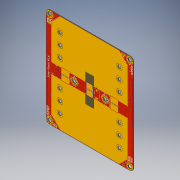
# Autodesk Inventor part: SolarPanel_PCB
Saved by Autodesk Inventor 2018 (Build 220112000, 112)
## iProperties
Created: 2018-11-29
Part Number: SolarPanel_PCB
Material: Epoxy Resin
Document SubType Name: Modeling
Designer: Bradley
Density: 1.14 g/cm^3
Appearance: Smooth - Dark Gray
Author: Bradley
Autodesk Inventor part; units mm, degrees
ref_plane "YZ Plane" through (0, 0, 0) normal (1, 0, 0) x (0, 1, 0)
ref_plane "XZ Plane" through (0, 0, 0) normal (0, 1, 0) x (-1, 0, 0)
ref_plane "XY Plane" through (0, 0, 0) normal (0, 0, 1) x (1, 0, 0)
sketch "Sketch1" plane through (0, 0, 0) normal (0, 1, 0) x (-1, 0, 0)
  line L0 (36.5, -45) -> (-36.5, -45)
  line L1 (-39.5, -42) -> (-39.5, 42)
  line L2 (-36.5, 45) -> (36.5, 45)
  line L3 (39.5, 42) -> (39.5, -42)
  line L4 (39.5, -45) -> (-39.5, 45) construction
  line L5 (-39.5, -45) -> (39.5, 45) construction
  arc A0 (39.5, 42) -> (36.5, 45) centre (36.5, 42) ccw
  arc A1 (36.5, -45) -> (39.5, -42) centre (36.5, -42) ccw
  arc A2 (-39.5, -42) -> (-36.5, -45) centre (-36.5, -42) ccw
  arc A3 (-36.5, 45) -> (-39.5, 42) centre (-36.5, 42) ccw
  circle A4 centre (36.5, 42) radius 1.65
  circle A5 centre (-36.5, 42) radius 1.65
  circle A6 centre (-36.5, -42) radius 1.65
  circle A7 centre (36.5, -42) radius 1.65
  line L6 (14, 0) -> (-14, 0) construction
  circle A8 centre (14, 0) radius 1.65
  circle A9 centre (-14, 0) radius 1.65
  point P0 (0, 0)
  point P1 (0, 0)
  dimension "d0" = 79
  dimension "d1" = 90
  dimension "d2" = 3
  dimension "d3" = 3.3
  dimension "d4" = 28
  constraints: 14 end point, 10 centre point, 8 equal radius, 8 point on circle, 8 point on line, 8 tangent, 6 coincident, 4 midpoint, 2 horizontal, 2 parallel, 1 perpendicular
  measures "d0" distance of L4.end L5.end
  measures "d1" distance of L5.end L4.start
  measures "d2" radius of A0
  measures "d3" diameter of A4
  measures "d4" distance of L6.start L6.end
extrude "Extrusion1" add sketch "Sketch1" along normal mid plane 0.6
sketch "Sketch2" plane through (0, -0.3, 0) normal (0, -1, 0) x (1, 0, 0)
  circle A0 centre (14, 0) radius 1.65 projected
  circle A1 centre (-14, 0) radius 1.65 projected
  circle A2 centre (-36.5, -42) radius 1.65 projected
  circle A3 centre (36.5, -42) radius 1.65 projected
  circle A4 centre (36.5, 42) radius 1.65 projected
  circle A5 centre (-36.5, 42) radius 1.65 projected
  line L0 (-39.5, 42) -> (-39.5, -42) projected
  arc A6 (-39.5, -42) -> (-36.5, -45) centre (-36.5, -42) ccw projected
  line L1 (-36.5, -45) -> (36.5, -45) projected
  arc A7 (36.5, -45) -> (39.5, -42) centre (36.5, -42) ccw projected
  line L2 (39.5, -42) -> (39.5, 42) projected
  arc A8 (39.5, 42) -> (36.5, 45) centre (36.5, 42) ccw projected
  line L3 (36.5, 45) -> (-36.5, 45) projected
  arc A9 (-36.5, 45) -> (-39.5, 42) centre (-36.5, 42) ccw projected
  line L4 (-39.5, 42) -> (-39.5, -42) projected
  line L5 (39.5, -42) -> (39.5, 42) projected
  line L6 (-39.5, 44.9931) -> (39.5, 44.9931) construction
  line L7 (39.5, 44.9931) -> (39.5, -44.9931) construction
  line L8 (39.5, -44.9931) -> (-39.5, -44.9931) construction
  line L9 (-39.5, -44.9931) -> (-39.5, 44.9931) construction
  point P0 (0, 0)
  point P1 (39.5, 0)
  point P2 (39.5, 0)
  point P3 (39.5, 0)
  point P4 (39.5, 0)
  point P5 (39.5, 0)
  point P6 (39.5, 0)
  constraints: 7 midpoint, 2 collinear, 2 other
decal "Decal1"
sketch "Sketch3" plane through (0, 0.3, 0) normal (0, 1, 0) x (1, 0, 0)
  circle A0 centre (14, 0) radius 1.65 projected
  circle A1 centre (-14, 0) radius 1.65 projected
  circle A2 centre (-36.5, 42) radius 1.65 projected
  circle A3 centre (36.5, 42) radius 1.65 projected
  circle A4 centre (36.5, -42) radius 1.65 projected
  circle A5 centre (-36.5, -42) radius 1.65 projected
  line L0 (-39.5, 42) -> (-39.5, -42) projected
  arc A6 (-39.5, -42) -> (-36.5, -45) centre (-36.5, -42) ccw projected
  line L1 (-36.5, -45) -> (36.5, -45) projected
  arc A7 (36.5, -45) -> (39.5, -42) centre (36.5, -42) ccw projected
  line L2 (39.5, -42) -> (39.5, 42) projected
  arc A8 (39.5, 42) -> (36.5, 45) centre (36.5, 42) ccw projected
  line L3 (36.5, 45) -> (-36.5, 45) projected
  arc A9 (-36.5, 45) -> (-39.5, 42) centre (-36.5, 42) ccw projected
  line L4 (39.5, -42) -> (39.5, 42) projected
  line L5 (39.5, -44.9829) -> (-39.5, -44.9829) construction
  line L6 (-39.5, -44.9829) -> (-39.5, 44.9829) construction
  line L7 (-39.5, 44.9829) -> (39.5, 44.9829) construction
  line L8 (39.5, 44.9829) -> (39.5, -44.9829) construction
  point P0 (0, 0)
  point P1 (39.5, 0)
  point P2 (39.5, 0)
  point P3 (39.5, 0)
  point P4 (39.5, 0)
  point P5 (39.5, 0)
  constraints: 6 midpoint, 2 collinear, 2 other
decal "Decal2"
sketch "Sketch4" plane through (0, -0.3, 0) normal (0, -1, 0) x (1, 0, 0)
  point P0 (0, 0)
  point P1 (27, -22)
  point P2 (27, 32)
  point P3 (27, 22)
  point P4 (27, 12)
  point P5 (-27, 32)
  point P6 (27, -12)
  point P7 (-27, 22)
  point P8 (-27, 12)
  point P9 (-27, -32)
  point P10 (-27, -22)
  point P11 (27, -32)
  point P12 (-27, -12)
  constraints: 12 other
hole "Hole1" at (27, -0.3, -22) at (27, -0.3, 32) at (27, -0.3, 22) at (27, -0.3, 12) at (-27, -0.3, 32) at (27, -0.3, -12) at (-27, -0.3, 22) at (-27, -0.3, 12) at (-27, -0.3, -32) at (-27, -0.3, -22) at (27, -0.3, -32) at (-27, -0.3, -12) direction (0, 1, 0) diameter 3 end through all
sketch "Sketch5" plane through (0, -0.3, 0) normal (0, -1, 0) x (1, 0, 0)
  point P0 (0, 0)
  point P1 (-12.374, -1.626)
  point P2 (-15.626, -1.626)
  point P3 (-14, -2.3)
  point P4 (-15.626, 1.626)
  point P5 (-14, 2.3)
  point P6 (-12.374, 1.626)
  point P7 (-11.7, 0)
  point P8 (-16.3, 0)
  point P9 (34.874, -40.374)
  point P10 (38.126, -43.626)
  point P11 (34.874, -43.626)
  point P12 (36.5, -39.7)
  point P13 (38.126, -40.374)
  point P14 (38.8, -42)
  point P15 (34.2, -42)
  point P16 (36.5, -44.3)
  point P17 (34.874, 40.374)
  point P18 (36.5, 39.7)
  point P19 (34.874, 43.626)
  point P20 (36.5, 44.3)
  point P21 (38.126, 43.626)
  point P22 (38.8, 42)
  point P23 (34.2, 42)
  point P24 (38.126, 40.374)
  point P25 (-34.874, 40.374)
  point P26 (-38.126, 40.374)
  point P27 (-36.5, 39.7)
  point P28 (-38.126, 43.626)
  point P29 (-36.5, 44.3)
  point P30 (-34.874, 43.626)
  point P31 (-34.2, 42)
  point P32 (15.626, -1.626)
  point P33 (12.374, -1.626)
  point P34 (-34.874, -43.626)
  point P35 (14, -2.3)
  point P36 (12.374, 1.626)
  point P37 (14, 2.3)
  point P38 (15.626, 1.626)
  point P39 (-38.126, -43.626)
  point P40 (-38.8, 42)
  point P41 (-38.126, -40.374)
  point P42 (-36.5, -39.7)
  point P43 (-34.874, -40.374)
  point P44 (-34.2, -42)
  point P45 (-38.8, -42)
  point P46 (16.3, 0)
  point P47 (11.7, 0)
  point P48 (-36.5, -44.3)
  constraints: 48 other
hole "Hole2" at (-12.374, -0.3, -1.626) at (-15.626, -0.3, -1.626) at (-14, -0.3, -2.3) at (-15.626, -0.3, 1.626) at (-14, -0.3, 2.3) at (-12.374, -0.3, 1.626) at (-11.7, -0.3, 0) at (-16.3, -0.3, 0) at (34.874, -0.3, -40.374) at (38.126, -0.3, -43.626) at (34.874, -0.3, -43.626) at (36.5, -0.3, -39.7) at (38.126, -0.3, -40.374) at (38.8, -0.3, -42) at (34.2, -0.3, -42) at (36.5, -0.3, -44.3) at (34.874, -0.3, 40.374) at (36.5, -0.3, 39.7) at (34.874, -0.3, 43.626) at (36.5, -0.3, 44.3) at (38.126, -0.3, 43.626) at (38.8, -0.3, 42) at (34.2, -0.3, 42) at (38.126, -0.3, 40.374) at (-34.874, -0.3, 40.374) at (-38.126, -0.3, 40.374) at (-36.5, -0.3, 39.7) at (-38.126, -0.3, 43.626) at (-36.5, -0.3, 44.3) at (-34.874, -0.3, 43.626) at (-34.2, -0.3, 42) at (15.626, -0.3, -1.626) at (12.374, -0.3, -1.626) at (-34.874, -0.3, -43.626) at (14, -0.3, -2.3) at (12.374, -0.3, 1.626) at (14, -0.3, 2.3) at (15.626, -0.3, 1.626) at (-38.126, -0.3, -43.626) at (-38.8, -0.3, 42) at (-38.126, -0.3, -40.374) at (-36.5, -0.3, -39.7) at (-34.874, -0.3, -40.374) at (-34.2, -0.3, -42) at (-38.8, -0.3, -42) at (16.3, -0.3, 0) at (11.7, -0.3, 0) at (-36.5, -0.3, -44.3) direction (0, 1, 0) diameter 0.45 end through all
sketch "Sketch6" plane through (0, -0.3, 0) normal (0, -1, 0) x (1, 0, 0)
  point P0 (0, 0)
  point P1 (26.235, 1.5)
  point P2 (2.985, 2.5)
  point P3 (6.035, -1.035)
  point P4 (6.035, 0.535)
  point P5 (4.465, -1.25)
  point P6 (31.8, 40.1)
  point P7 (38.875, -9.597)
  point P8 (-26.245, -4)
  point P9 (37.454, 17.611)
  point P10 (8.75, 4.5)
  point P11 (2.985, 3.44)
  point P12 (35, 33.69)
  point P13 (35, 5)
  point P14 (10, -4)
  point P15 (4.465, -2.06)
  point P16 (23.01, 0)
  point P17 (-31.656, 2.294)
  point P18 (-36.638, 33.75)
  point P19 (-36.745, -3.622)
  point P20 (-26.26, -0.6)
  point P21 (8.708, -2.792)
  point P22 (8.01, 2.75)
  point P23 (35.479, 3.859)
  point P24 (37, 21.419)
  point P25 (37.5, -8.585)
  point P26 (37.113, 15.25)
  point P27 (37.165, 6.415)
  point P28 (37.78, 29.372)
  point P29 (37.165, 3.962)
  point P30 (0, 0)
  point P31 (13.555, -4.25)
  point P32 (18.25, -4.25)
  point P33 (26, -1.5)
  point P34 (36.38, 9.38)
  point P35 (7.25, -0.25)
  point P36 (-35.75, 33.75)
  point P37 (4.465, 1.635)
  point P38 (-27.765, 1.065)
  point P39 (-32, 3.6)
  point P40 (-26.081, 2.75)
  point P41 (-27.79, -4)
  point P42 (-34.44, 3.458)
  point P43 (-30, -3.915)
  point P44 (-34.44, 4.25)
  point P45 (-29.321, -3.448)
  point P46 (-35.313, -17.51)
  point P47 (-35.223, 8.473)
  point P48 (-35, -16.75)
  point P49 (-35, 7.5)
  point P50 (2.985, 4.25)
  point P51 (6.035, 4.523)
  point P52 (35.039, 35.789)
  point P53 (35.945, 8.67)
  point P54 (35.585, 7.5)
  point P55 (35, 35)
  point P56 (-3.015, -2.188)
  point P57 (-10.155, -2.25)
  point P58 (-11.534, -2.466)
  point P59 (-33.855, -2.895)
  point P60 (-34.415, 0.4)
  point P61 (36.64, 14.648)
  point P62 (36.64, 12.516)
  point P63 (37.789, 31)
  point P64 (3, -0.785)
  point P65 (3, -4)
  point P66 (-36.145, -5.186)
  point P67 (-26.233, -2.233)
  point P68 (-28.544, 4.544)
  point P69 (-18.25, 0.75)
  point P70 (-35.943, 9.846)
  point P71 (37.085, 32.75)
  point P72 (-34.415, 1.25)
  point P73 (-32.466, 0.657)
  point P74 (-28.565, -0.585)
  point P75 (-9.595, 3.75)
  point P76 (36.885, 24.5)
  point P77 (-26.21, -1.473)
  point P78 (-17.9, 3)
  point P79 (-26.26, 0.2)
  point P80 (-36.12, -2.812)
  point P81 (-33.4, -0.3)
  point P82 (-30.9, -1)
  point P83 (-29.253, 0.647)
  point P84 (11.75, 3.5)
  point P85 (18.25, 3.5)
  point P86 (36.039, 5.211)
  point P87 (36.039, -3.228)
  point P88 (37.252, -10.392)
  point P89 (37, 13.888)
  point P90 (35.047, 38.56)
  constraints: 90 other
hole "Hole3" at (35.047, -0.3, 38.56) at (37, -0.3, 13.888) at (37.252, -0.3, -10.392) at (36.039, -0.3, -3.228) at (36.039, -0.3, 5.211) at (18.25, -0.3, 3.5) at (11.75, -0.3, 3.5) at (36.885, -0.3, 24.5) at (37.085, -0.3, 32.75) at (3, -0.3, -4) at (3, -0.3, -0.785) at (37.789, -0.3, 31) at (36.64, -0.3, 12.516) at (36.64, -0.3, 14.648) at (35, -0.3, 35) at (35.585, -0.3, 7.5) at (35.945, -0.3, 8.67) at (35.039, -0.3, 35.789) at (6.035, -0.3, 4.523) at (2.985, -0.3, 4.25) at (4.465, -0.3, 1.635) at (7.25, -0.3, -0.25) at (36.38, -0.3, 9.38) at (26, -0.3, -1.5) at (18.25, -0.3, -4.25) at (13.555, -0.3, -4.25) at (0, -0.3, 0) at (37.165, -0.3, 3.962) at (37.78, -0.3, 29.372) at (37.165, -0.3, 6.415) at (37.113, -0.3, 15.25) at (37.5, -0.3, -8.585) at (37, -0.3, 21.419) at (35.479, -0.3, 3.859) at (8.01, -0.3, 2.75) at (8.708, -0.3, -2.792) at (23.01, -0.3, 0) at (4.465, -0.3, -2.06) at (10, -0.3, -4) at (35, -0.3, 5) at (35, -0.3, 33.69) at (2.985, -0.3, 3.44) at (8.75, -0.3, 4.5) at (37.454, -0.3, 17.611) at (38.875, -0.3, -9.597) at (31.8, -0.3, 40.1) at (4.465, -0.3, -1.25) at (6.035, -0.3, 0.535) at (6.035, -0.3, -1.035) at (2.985, -0.3, 2.5) direction (0, 1, 0) diameter 0.3 end through all and at (26.235, -0.3, 1.5) (-29.253, -0.3, 0.647) (-30.9, -0.3, -1) (-33.4, -0.3, -0.3) (-36.12, -0.3, -2.812) (-26.26, -0.3, 0.2) (-17.9, -0.3, 3) (-26.21, -0.3, -1.473) (-9.595, -0.3, 3.75) (-28.565, -0.3, -0.585) (-32.466, -0.3, 0.657) (-34.415, -0.3, 1.25) (-35.943, -0.3, 9.846) (-18.25, -0.3, 0.75) (-28.544, -0.3, 4.544) (-26.233, -0.3, -2.233) (-36.145, -0.3, -5.186) (-34.415, -0.3, 0.4) (-33.855, -0.3, -2.895) (-11.534, -0.3, -2.466) (-10.155, -0.3, -2.25) (-35, -0.3, 7.5) (-35, -0.3, -16.75) (-35.223, -0.3, 8.473) (-35.313, -0.3, -17.51) (-29.321, -0.3, -3.448) (-34.44, -0.3, 4.25) (-30, -0.3, -3.915) (-34.44, -0.3, 3.458) (-27.79, -0.3, -4) (-26.081, -0.3, 2.75) (-32, -0.3, 3.6) (-27.765, -0.3, 1.065) (-35.75, -0.3, 33.75) (-26.26, -0.3, -0.6) (-36.745, -0.3, -3.622) (-36.638, -0.3, 33.75) (-31.656, -0.3, 2.294) (-26.245, -0.3, -4) (-3.015, -0.3, -2.188)
sketch "Sketch7" plane through (0, -0.3, 0) normal (0, -1, 0) x (1, 0, 0)
  point P0 (0, 0)
  point P1 (-11.8, 4.335)
  point P2 (-28.434, 1.507)
  point P3 (-35.747, -21.447)
  point P4 (-35, -25.3)
  point P5 (-36.318, -19.054)
  point P6 (-35.02, -24.4)
  point P7 (-30.1, -42.2)
  point P8 (-27.595, 2.345)
  point P9 (-29.3, -42.9)
  constraints: 9 other
hole "Hole4" at (-11.8, -0.3, 4.335) at (-28.434, -0.3, 1.507) at (-35.747, -0.3, -21.447) at (-35, -0.3, -25.3) at (-36.318, -0.3, -19.054) at (-35.02, -0.3, -24.4) at (-30.1, -0.3, -42.2) at (-27.595, -0.3, 2.345) at (-29.3, -0.3, -42.9) direction (0, 1, 0) diameter 0.35 end through all
body "Solid1"
